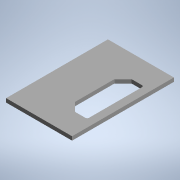
# Autodesk Inventor part: P002-Cache-HDMI
Saved by Autodesk Inventor 2020 (Build 240168000, 168)
## iProperties
Created: 2021-07-23
Part Number: P002-Cache-HDMI
Material: Générique
Document SubType Name: Modeling
Designer: gregory.trottet
Density: 1 g/cm^3
Appearance: Par défaut
Author: gregory.trottet
Autodesk Inventor part; units mm, degrees
ref_plane "YZ Plane" through (0, 0, 0) normal (1, 0, 0) x (0, 1, 0)
ref_plane "XZ Plane" through (0, 0, 0) normal (0, 1, 0) x (-1, 0, 0)
ref_plane "XY Plane" through (0, 0, 0) normal (0, 0, 1) x (1, 0, 0)
sketch "Sketch1" plane through (0, 0, 0) normal (0, 0, 1) x (1, 0, 0)
  line L0 (5, 7.5) -> (2.5, 7.5)
  line L1 (0, 5) -> (0, -5)
  line L2 (2.5, -7.5) -> (5, -7.5)
  line L3 (5.5, -7) -> (5.5, 7)
  line L4 (2.1464, 7.3536) -> (0.1464, 5.3536)
  line L5 (2.1464, -7.3536) -> (0.1464, -5.3536)
  line L6 (5.5, 0) -> (-0.5, 0) construction
  arc A0 (5.5, 7) -> (5, 7.5) centre (5, 7) ccw
  arc A1 (5, -7.5) -> (5.5, -7) centre (5, -7) ccw
  arc A2 (2.1464, -7.3536) -> (2.5, -7.5) centre (2.5, -7) ccw
  arc A3 (0, -5) -> (0.1464, -5.3536) centre (0.5, -5) ccw
  arc A4 (0.1464, 5.3536) -> (0, 5) centre (0.5, 5) ccw
  arc A5 (2.5, 7.5) -> (2.1464, 7.3536) centre (2.5, 7) ccw
  line L7 (5, 7) -> (5, -7)
  line L8 (5, -7) -> (2.5, -7)
  line L9 (2.5, -7) -> (0.5, -5)
  line L10 (0.5, -5) -> (0.5, 5)
  line L11 (0.5, 5) -> (2.5, 7)
  line L12 (2.5, 7) -> (5, 7)
  line L13 (7.5, 13.5) -> (-10, 13.5)
  line L14 (-10, 13.5) -> (-10, -13.5)
  line L15 (-10, -13.5) -> (7.5, -13.5)
  line L16 (7.5, -13.5) -> (7.5, 13.5)
  line L17 (5.5, 0) -> (7.5, 0) construction
  point P0 (0, 0)
  point P1 (-0.5, 0)
  point P2 (5.5, 7.5)
  point P3 (5.5, -7.5)
  point P4 (-0.5, 0)
  point P5 (0, 0)
  dimension "d0" = 0.5
  dimension "d1" = 15
  dimension "d2" = 5.5
  dimension "d3" = 0.5
  dimension "d4" = 135
  dimension "d5" = 3
  dimension "d6" = 0.5
  dimension "d7" = 10
  dimension "d8" = 27
  dimension "d9" = 2
  constraints: 36 end point, 12 point on circle, 12 tangent, 6 centre point, 6 parallel, 5 equal radius, 5 point on line, 4 horizontal, 4 perpendicular, 3 midpoint, 1 coincident, 9 other
  measures "d1" distance of point (5.5, -7.5) point (5.5, 7.5)
  measures "d2" distance between parallel lines of L3 L1
  measures "d3" radius of A0
  measures "d4" angle of L0 L4
  measures "d5" distance from line of L2.start L3
  measures "d6" distance between parallel lines of L3 L7
  measures "d7" distance between parallel lines of L14 L1
  measures "d8" distance of L15.end L13.start
  measures "d9" distance between parallel lines of L3 L16
extrude "Extrusion1" add sketch "Sketch1" along normal blind 1 contours L16 L15 L14 L13
body "Solid1"
